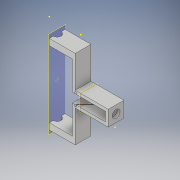
# Autodesk Inventor part: Neue Grundplatte
Saved by Autodesk Inventor 2018.3 (Build 223284000, 284)
## iProperties
Created: 2018-10-25
Part Number: Neue Grundplatte
Material: Generisch
Document SubType Name: Modeling
Designer: pgmadmin
Density: 1 g/cm^3
Appearance: Vorgabe
Author: pgmadmin
Autodesk Inventor part; units mm, degrees
ref_plane "YZ Plane" through (0, 0, 0) normal (1, 0, 0) x (0, 1, 0)
ref_plane "XZ Plane" through (0, 0, 0) normal (0, 1, 0) x (-1, 0, 0)
ref_plane "XY Plane" through (0, 0, 0) normal (0, 0, 1) x (1, 0, 0)
sketch "Skizze1" plane through (0, 0, 0) normal (0, 1, 0) x (-1, 0, 0)
  line L0 (50.5762, -64.7123) -> (8.5762, -64.7123)
  line L1 (8.5762, -64.7123) -> (8.5762, -84.3623)
  line L2 (8.5762, -84.3623) -> (50.5762, -84.3623)
  line L3 (54.0762, -68.7123) -> (54.0762, -32.0373)
  line L4 (54.0762, -32.0373) -> (108.5762, -32.0373)
  line L5 (108.5762, -32.0373) -> (108.5762, -24.0373)
  line L6 (108.5762, -24.0373) -> (50.5762, -24.0373)
  line L7 (50.5762, -24.0373) -> (50.5762, -64.7123)
  line L8 (54.0762, -117.0373) -> (108.5762, -117.0373)
  line L9 (108.5762, -117.0373) -> (108.5762, -125.0373)
  line L10 (108.5762, -125.0373) -> (50.5762, -125.0373)
  line L11 (50.5762, -125.0373) -> (50.5762, -84.3623)
  line L12 (54.0762, -80.3623) -> (54.0762, -117.0373)
  line L13 (12.0762, -68.7123) -> (12.0762, -80.3623)
  line L14 (12.0762, -68.7123) -> (54.0762, -68.7123)
  line L15 (54.0762, -80.3623) -> (12.0762, -80.3623)
  point P0 (0, 0)
  dimension "d1" = 8
  dimension "d2" = 3.5
  dimension "d5" = 8
  dimension "d9" = 4
  dimension "d10" = 100
  dimension "d11" = 11.65
  dimension "d27" = 3.5
  dimension "d29" = 42
  dimension "d30" = 85
  dimension "d31" = 36.675
  constraints: 32 end point, 9 perpendicular, 5 point on line, 1 horizontal, 1 parallel
  measures "d1" distance between parallel lines of L10 L8
  measures "d2" distance between parallel lines of L11 L12
  measures "d5" distance between parallel lines of L6 L4
  measures "d9" distance between parallel lines of L2 L15
  measures "d10" distance between parallel lines of L9 L1
  measures "d11" distance between parallel lines of L15 L14
  measures "d27" distance between parallel lines of L13 L1
  measures "d29" distance between parallel lines of L1 L7
  measures "d30" distance between parallel lines of L8 L4
  measures "d31" distance between parallel lines of L14 L4
extrude "Extrusion1" add sketch "Skizze1" along normal blind 20
sketch "Skizze3" plane through (-12.0762, 0, -68.7123) normal (0, 0, -1) x (-1, 0, 0)
  line L0 (39, 0) -> (23.696, 15.304)
  line L1 (37.5, 0) -> (22.946, 14.554)
  line L2 (22.946, 14.554) -> (23.696, 15.304)
  line L3 (42, 0) -> (42, 20) projected
  line L4 (42, -13) -> (42, 0)
  line L5 (37.5, 0) -> (39, 0)
  line L6 (0, 0) -> (42, 0) projected
  point P0 (-12.0762, 0)
  point P1 (-3.5, 0)
  dimension "d19" = 1.5
  dimension "d21" = 15.304
  dimension "d26" = 41
  constraints: 10 end point, 2 collinear, 2 point on line, 1 perpendicular
  measures "d19" distance of L0.start L1.start
  measures "d21" horizontal distance of L0.start L0.end
  measures "d26" distance of point (-3.5, 0) L1.start
extrude "Extrusion3" cut sketch "Skizze3" against normal blind 2.5
sketch "Skizze4" plane through (-108.5762, 0, -24.0373) normal (0, 0, 1) x (1, 0, 0)
  line L0 (0, 0) -> (0, 20) projected
  circle A0 centre (0, 10) radius 5
  point P0 (108.5762, 0)
  dimension "d32" = 10
  constraints: 1 centre point, 1 coincident, 1 midpoint
  measures "d32" diameter of A0
extrude "Extrusion4" cut sketch "Skizze4" against normal blind 200
sketch "Skizze5" plane through (-54.0762, 0, -80.3623) normal (0, 0, 1) x (1, 0, 0)
  point P0 (54.0762, 0)
sketch "Skizze6" plane through (-54.0762, 0, -80.3623) normal (0, 0, 1) x (1, 0, 0)
  line L0 (0, 0) -> (42, 0) projected
  line L1 (4.5, 0) -> (19.804, 15.304)
  line L2 (19.804, 15.304) -> (19.8768, 16.8022)
  line L3 (19.8768, 16.8022) -> (3, 0)
  line L4 (0, 0) -> (0, -2.9867)
  line L5 (4.5, 0) -> (0, 0)
  point P0 (54.0762, 0)
  point P1 (45.5, 0)
  dimension "d35" = 45
  dimension "d36" = 15.304
  dimension "d37" = 1.5
  dimension "d38" = 1.5
  dimension "d39" = 41
  constraints: 10 end point, 3 point on line, 1 collinear, 1 vertical
  measures "d35" angle of L1 L0
  measures "d36" horizontal distance of L1.start L1.end
  measures "d37" distance of L1.end L2.end
  measures "d38" distance of L3.end L1.start
  measures "d39" distance of point (45.5, 0) L1.start
extrude "Extrusion5" cut sketch "Skizze6" against normal blind 2.5
sketch "Skizze7" plane through (-108.5762, 20, -32.0373) normal (-1, 0, 0) x (0, 0, 1)
  line L0 (8, -5) -> (8, 0) projected
  line L1 (8, -15) -> (0, -15) projected
  line L2 (0, -5) -> (8, -5) projected
  line L3 (-93, -5) -> (-93, 0) projected
  point P0 (32.0373, -20)
  point P1 (4, -2.5)
  point P2 (3.7984, -17.5)
  point P3 (-89, -2.5)
  point P4 (-89, -17.5)
  dimension "d42" = 4
  dimension "d43" = 2.5
  dimension "d44" = 2.5
  dimension "d52" = 4
  measures "d42" distance from line of L0 point (4, -2.5)
  measures "d43" distance from line of L1 point (3.798, -17.5)
  measures "d44" distance from line of L2 point (4, -2.5)
  measures "d52" distance from line of point (-89, -2.5) L3
hole "Bohrung1" at (-108.5762, 17.5, -28.0373) at (-108.5762, 2.5, -28.2389) direction (1, 0, 0) diameter 2.75 depth 8 tip angle 118
sketch "Skizze8" plane through (-108.5762, 0, -125.0373) normal (-1, 0, 0) x (0, 0, 1)
  line L0 (8, 15) -> (8, 20) projected
  line L1 (0, 20) -> (8, 20) projected
  line L2 (0, 0) -> (8, 0) projected
  point P0 (125.0373, 0)
  point P1 (4, 17.5)
  point P2 (3.9503, 2.5)
  dimension "d53" = 4
  dimension "d54" = 2.5
  dimension "d55" = 2.5
  measures "d53" distance from line of L0 point (4, 17.5)
  measures "d54" distance from line of L1 point (4, 17.5)
  measures "d55" distance from line of L2 point (3.95, 2.5)
hole "Bohrung2" at (-108.5762, 2.5, -121.087) at (-108.5762, 17.5, -121.0373) direction (1, 0, 0) diameter 2.75 depth 8 tip angle 118
sketch "Skizze9" plane through (-8.5762, 0, -64.7123) normal (1, 0, 0) x (0, 0, -1)
  line L0 (0, 0) -> (0, 20) projected
  line L1 (0, 0) -> (19.65, 0) projected
  point P0 (-64.7123, 0)
  point P1 (10, 10)
  dimension "d63" = 10
  dimension "d64" = 10
  measures "d63" distance from line of point (10, 10) L0
  measures "d64" distance from line of L1 point (10, 10)
hole "Bohrung3" at (-8.5762, 10, -74.7123) direction (-1, 0, 0) diameter 10 depth 5 tip angle 118
sketch "Skizze12" plane through (-108.5762, 0, -24.0373) normal (0, 0, 1) x (1, 0, 0)
  line L0 (58, 20) -> (0, 20) projected
  line L1 (0, 0) -> (25, 0)
  line L2 (25, 0) -> (25, 20)
  line L3 (25, 20) -> (0, 20)
  line L4 (0, 20) -> (0, 0)
  point P0 (108.5762, 0)
  dimension "d75" = 25
  dimension "d76" = 20
  constraints: 8 end point, 2 parallel, 1 horizontal, 1 perpendicular, 1 point on line
  measures "d75" distance of L1.start L1.end
  measures "d76" distance of L1.end L2.end
extrude "Extrusion6" cut sketch "Skizze12" against normal blind 120
sketch "Skizze13" plane through (-50.5762, 0, -24.0373) normal (0, 0, 1) x (1, 0, 0)
  line L0 (-33, 0) -> (-33, 20) projected
  circle A0 centre (-33, 10) radius 5
  point P0 (50.5762, 0)
  dimension "d79" = 10
  constraints: 1 centre point, 1 coincident, 1 midpoint
  measures "d79" diameter of A0
extrude "Extrusion7" cut sketch "Skizze13" against normal blind 120
sketch "Skizze14" plane through (-83.5762, 0, -32.0373) normal (-1, 0, 0) x (0, 0, 1)
  line L0 (8, 5) -> (0, 5) projected
  line L1 (0, 0) -> (0, 5) projected
  line L2 (0, 20) -> (8, 20) projected
  line L3 (8, 20) -> (8, 15) projected
  line L4 (-85, 5) -> (-93, 5) projected
  line L5 (-85, 5) -> (-85, 0) projected
  line L6 (-93, 20) -> (-85, 20) projected
  line L7 (-85, 20) -> (-85, 15) projected
  point P0 (32.0373, 0)
  point P1 (4, 2.5)
  point P2 (4, 17.5)
  point P3 (-89, 2.5)
  point P4 (-89, 17.5)
  dimension "d82" = 2.5
  dimension "d83" = 4
  dimension "d84" = 2.5
  dimension "d85" = 4
  dimension "d86" = 2.5
  dimension "d87" = 4
  dimension "d88" = 2.5
  dimension "d89" = 4
  measures "d82" distance from line of L0 point (4, 2.5)
  measures "d83" distance from line of L1 point (4, 2.5)
  measures "d84" distance from line of L2 point (4, 17.5)
  measures "d85" distance from line of L3 point (4, 17.5)
  measures "d86" distance from line of L4 point (-89, 2.5)
  measures "d87" distance from line of L5 point (-89, 2.5)
  measures "d88" distance from line of L6 point (-89, 17.5)
  measures "d89" distance from line of L7 point (-89, 17.5)
hole "Bohrung4" at (-83.5762, 2.5, -28.0373) at (-83.5762, 17.5, -28.0373) at (-83.5762, 17.5, -121.0373) at (-83.5762, 2.5, -121.0373) direction (1, 0, 0) diameter 3 depth 8 tip angle 118
ref_plane "Arbeitsebene3" through (-43.5762, 0, -64.7123) normal (1, 0, 0) x (0, 0, -1)
ref_plane "Arbeitsebene4" through (-83.5762, 17.5, -24.0373) normal (-1, 0, 0) x (0, 0, 1)
sketch "Skizze15" plane through (-83.5762, 17.5, -24.0373) normal (-1, 0, 0) x (0, 0, 1)
  point P0 (24.0373, -17.5)
  point P1 (-50.5568, -7.548)
sketch "Skizze16" plane through (-43.5762, 0, -64.7123) normal (1, 0, 0) x (0, 0, -1)
  point P0 (-64.7123, 0)
  point P1 (9.9474, 9.9802)
